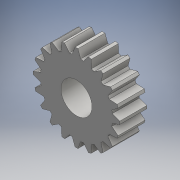
# Autodesk Inventor part: gear_small
Saved by Autodesk Inventor 2016 (Build 200138000, 138)
## iProperties
Created: 2015-10-28
Part Number: gear_small
Material: Gypsum Wall Board
Document SubType Name: Modeling
Designer: Meet
Density: 1.1 g/cm^3
Appearance: Gypsum Board - Painted White
Author: Meet
Autodesk Inventor part; units mm, degrees
ref_plane "YZ Plane" through (0, 0, 0) normal (1, 0, 0) x (0, 1, 0)
ref_plane "XZ Plane" through (0, 0, 0) normal (0, 1, 0) x (-1, 0, 0)
ref_plane "XY Plane" through (0, 0, 0) normal (0, 0, 1) x (1, 0, 0)
sketch "Sketch1" plane through (0, 0, 0) normal (0, 1, 0) x (-1, 0, 0)
  arc A0 (19.8614, 2.3507) -> (19.8614, -2.3507) centre (0, 0) ccw
  arc A1 (23.9872, -0.7853) -> (23.9872, 0.7853) centre (0, 0) ccw
  line L0 (0, 0) -> (20, 0) construction
  line L1 (0, 0) -> (24, 0) construction
  line L2 (23.9872, -0.7853) -> (19.8614, -2.3507)
  line L3 (23.9872, 0.7853) -> (19.8614, 2.3507)
  constraints: 8 end point, 4 point on circle, 2 centre point, 2 coincident, 2 horizontal, 2 symmetric about line, 1 point on line
extrude "Extrusion1" add sketch "Sketch1" along normal blind 15
pattern_circular "Circular Pattern1" count 20 over 360 about axis through (0, 0, 0) along (0, 1, 0) of "Extrusion1"
sketch "Sketch2" plane through (0, 0, 0) normal (0, -1, 0) x (1, 0, 0)
  circle A0 centre (0, 0) radius 8.6
  constraints: 1 centre point, 1 coincident
extrude "Extrusion2" cut sketch "Sketch2" against normal blind 15
body "Solid1"
